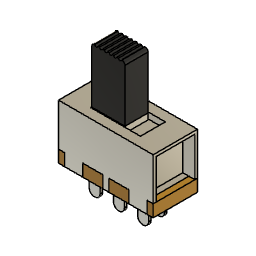
Slide_Switch_SS22F25-G7_ (Autodesk Fusion 360 design; units mm, degrees)
Autodesk Fusion 360 part; units mm, degrees
sketch "Sketch1" plane through (0, 0, 0) normal (0, 1, 0) x (1, 0, 0)
  line L0 (0, 0) -> (15.6, 0)
  line L1 (15.6, 0) -> (15.6, -2)
  line L2 (0, -2) -> (0, 0)
  line L3 (15.6, -2) -> (15.6, -9)
  line L4 (15.6, -9) -> (0, -9)
  line L5 (0, -9) -> (0, -2)
  line L6 (0, -2) -> (1, -2)
  line L7 (1, -2) -> (1, 0)
  line L8 (1, 0) -> (0, 0)
  line L9 (0, 0) -> (0, -2)
  line L10 (15.6, -2) -> (14.6, -2)
  line L11 (14.6, -2) -> (14.6, 0)
  line L12 (14.6, 0) -> (15.6, 0)
  line L13 (15.6, 0) -> (15.6, -2)
  line L14 (11.6, -2) -> (11.6, 0)
  line L15 (11.6, 0) -> (14.6, 0)
  line L16 (14.6, 0) -> (14.6, -2)
  line L17 (4, -2) -> (4, 0)
  line L18 (4, 0) -> (1, 0)
  line L19 (1, 0) -> (1, -2)
  line L20 (7.8, -14) -> (7.8, 4) construction
  line L21 (1, -2) -> (0, -2)
  line L22 (0, -2) -> (1, -2)
  line L23 (15.6, -2) -> (14.6, -2)
  line L24 (14.6, -2) -> (15.6, -2)
  line L25 (8.3, -2) -> (8.3, 0)
  line L26 (8.3, 0) -> (7.3, 0)
  line L27 (7.3, 0) -> (7.3, -2)
  line L28 (4, -2) -> (7.3, -2)
  line L29 (8.3, -2) -> (11.6, -2)
  line L30 (11.6, -2) -> (8.3, -2)
  line L31 (7.3, -2) -> (4, -2)
  dimension "d2" = 2
  dimension "d3" = 15.6
  dimension "d4" = 7
  dimension "d5" = 1
  dimension "d6" = 1
  dimension "d7" = 2
  dimension "d8" = 3
  dimension "d9" = 2
  dimension "d10" = 3
  dimension "d11" = 2
  dimension "d12" = 7.8
  dimension "d13" = 1
  dimension "d14" = 2
  constraint horizontal L0
  constraint vertical L1
  constraint horizontal L23
  constraint vertical L2
  constraint coincident L0.start L2.end
  constraint horizontal L22
  constraint vertical L3
  constraint horizontal L4
  constraint vertical L5
  constraint horizontal L6
  constraint vertical L7
  constraint horizontal L8
  constraint vertical L9
  constraint coincident L0 L7.end
  constraint horizontal L10
  constraint vertical L11
  constraint horizontal L12
  constraint vertical L13
  constraint vertical L14
  constraint horizontal L15
  constraint vertical L16
  constraint vertical L17
  constraint horizontal L18
  constraint vertical L19
  constraint vertical L20
  constraint collinear L21 L23
  constraint collinear L22 L28
  constraint collinear L23 L30
  constraint collinear L24 L28
  constraint vertical L25
  constraint horizontal L26
  constraint vertical L27
  constraint coincident L27.end L30
  constraint collinear L28 L29
  constraint collinear L30 L31
  measures "d2" distance of L0.start L2.start
  measures "d3" distance of L2.start L1.end
  measures "d4" distance of L2.start L4.end
  measures "d5" distance of L2.start L6.end
  measures "d6" distance of L1.end L10.end
  measures "d7" distance of L1.end L0.end
  measures "d8" distance of L10.end L14.start
  measures "d9" distance of L10.end L11.end
  measures "d10" distance of L6.end L17.start
  measures "d11" distance of L6.end L7.end
  measures "d12" distance of L5 L20
  measures "d13" distance of L27.end L25.start
  measures "d14" distance of L27.end L26.end
extrude "Extrude1" add sketch "Sketch1" along normal blind 7.3 contours L0 L3 L4 L5 L6 L7 L10 L11 L14 L15 L16 L17 L18 L19 L21 L22 L23 L24 L25 L26 L27 L28 L29 L30 L31 makes body 1
extrude "Extrude2" add sketch "Sketch1" along normal blind 7.3 separate body contours L0 L2 L6 L7 L8 L9 L19 L21 L22 | L0 L17 L27 L28 L31 | L0 L14 L25 L29 L30 | L0 L1 L10 L11 L12 L13 L16 L23 L24 makes body 2 at (5.1, 2.4333, 0) makes body 3 at (9.4, 2.4333, 0) makes body 4 at (1, 2.4333, 1.3333) makes body 5 at (14.6, 2.4333, 1.3333)
sketch "Sketch2" plane through (0, 0, 9) normal (0, 0, 1) x (-1, 0, 0)
  line L0 (0, 0) -> (-15.6, 0)
  line L1 (-15.6, 0) -> (-15.6, -7.3)
  line L2 (-15.6, -7.3) -> (0, -7.3)
  line L3 (0, -7.3) -> (0, 0)
  line L4 (0, 0) -> (-15.6, -7.3) construction
  line L5 (-15.6, 0) -> (0, -7.3) construction
  line L6 (-11.9, -1.6) -> (-3.7, -1.6)
  line L7 (-3.7, -1.6) -> (-3.7, -5.7)
  line L8 (-3.7, -5.7) -> (-11.9, -5.7)
  line L9 (-11.9, -5.7) -> (-11.9, -1.6)
  line L10 (-11.9, -1.6) -> (-3.7, -5.7) construction
  line L11 (-3.7, -1.6) -> (-11.9, -5.7) construction
  line L12 (-3.7, -5.55) -> (-9.2, -5.55)
  line L13 (-9.2, -5.55) -> (-9.2, -1.75)
  line L14 (-9.2, -1.75) -> (-3.7, -1.75)
  line L15 (-3.7, -1.75) -> (-3.7, -5.55)
  line L16 (1.4148, -3.65) -> (-17, -3.65) construction
  line L17 (1.4148, -1.75) -> (-17, -1.75) construction
  line L18 (-3.7, -1.75) -> (-3.77, -1.75) construction
  point P0 (-7.8, -3.65)
  dimension "d19" = 8.2
  dimension "d20" = 4.1
  dimension "d21" = 5.5
  dimension "d22" = 3.8
  dimension "d23" = 1.9
  constraint coincident L0.start L3.end
  constraint coincident L1.end L2.start
  constraint coincident L0.end L1.start
  constraint coincident L2.end L3.start
  constraint horizontal L6
  constraint perpendicular L6 L7
  constraint parallel L6 L8
  constraint parallel L7 L9
  constraint coincident L10 P0
  constraint coincident L11 P0
  constraint midpoint L5 P0
  constraint horizontal L12
  constraint vertical L13
  constraint horizontal L14
  constraint vertical L15
  constraint perpendicular L1 L16
  constraint coincident L17 L14.end
  constraint coincident L7 L14.end
  constraint coincident L17 L18.end
  measures "d19" distance of L7.end L8.end
  measures "d20" distance of L6.end L7.end
  measures "d21" distance of L12.start L12.end
  measures "d22" distance of L12.start L14.end
extrude "Extrude3" add sketch "Sketch2" along normal blind 9.2 separate body contours L7 L12 L13 L14 L15 makes body 6
extrude "Extrude4" cut sketch "Sketch2" against normal blind 1 contours L6 L7 L8 L9 L12 L13 L14 bodies 1
fillet "Fillet1" radius 0.5 2 edges at (9.2, 3.65, 18.2) (3.7, 3.65, 18.2) on bodies 6
sketch "Sketch3" plane through (0, 1.75, 0) normal (0, -1, 0) x (1, 0, 0)
  arc A0 (4.2, 18.2) -> (3.7, 17.7) centre (4.2, 17.7) ccw
  line L0 (3.7, 17.7) -> (3.7, 9)
  line L1 (3.7, 9) -> (9.2, 9)
  line L2 (9.2, 9) -> (9.2, 17.7)
  arc A1 (9.2, 17.7) -> (8.7, 18.2) centre (8.7, 17.7) ccw
  line L3 (8.7, 18.2) -> (4.2, 18.2)
  circle A2 centre (4.5, 18.2) radius 0.25
  circle A3 centre (5.28, 18.2) radius 0.25
  circle A4 centre (6.06, 18.2) radius 0.25
  circle A5 centre (6.84, 18.2) radius 0.25
  circle A6 centre (7.62, 18.2) radius 0.25
  circle A7 centre (8.4, 18.2) radius 0.25
  dimension "d30" = 0.5
  dimension "d43" = 3.9
  dimension "d44" = 0
  constraint coincident L3 A2.centre
  measures "d30" diameter of A2
extrude "Extrude6" cut sketch "Sketch3" against normal blind 5 contours L3 A2 | L3 A3 | L3 A4 | L3 A7 | L3 A5 | L3 A6 picked at (4.5053, 18.1045) picked at (5.2853, 18.1045) picked at (6.0653, 18.1045) picked at (8.4053, 18.1045) picked at (6.8453, 18.1045) picked at (7.6253, 18.1045) bodies 6
sketch "Sketch4" plane through (15.6, 0, 0) normal (1, 0, 0) x (0, 1, 0)
  line L0 (0, 9) -> (0, 2)
  line L1 (0, 2) -> (7.3, 2)
  line L2 (7.3, 2) -> (7.3, 9)
  line L3 (7.3, 9) -> (0, 9)
  line L4 (0.5, 8.5) -> (6.8816, 8.5)
  line L5 (6.8816, 8.5) -> (6.8816, 2)
  line L6 (6.8816, 2) -> (0.5, 2)
  line L7 (0.5, 2) -> (0.5, 8.5)
  dimension "d47" = 6.5
  constraint horizontal L4
  constraint vertical L5
  constraint horizontal L6
  constraint vertical L7
  measures "d47" distance of L4.start L6.end
extrude "Extrude7" cut sketch "Sketch4" against normal blind 2 contours L1 L4 L5 L6 L7 bodies 1
sketch "Sketch5" plane through (0, 0, 0) normal (-1, 0, 0) x (0, -1, 0)
  line L0 (0, 2) -> (0, 9)
  line L1 (0, 9) -> (-7.3, 9)
  line L2 (-7.3, 9) -> (-7.3, 2)
  line L3 (-7.3, 2) -> (0, 2)
  line L4 (-0.5, 8.5) -> (-6.8462, 8.5)
  line L5 (-6.8462, 8.5) -> (-6.8462, 2)
  line L6 (-6.8462, 2) -> (-0.5, 2)
  line L7 (-0.5, 2) -> (-0.5, 8.5)
  dimension "d50" = 6.5
  constraint horizontal L4
  constraint vertical L5
  constraint horizontal L6
  constraint vertical L7
  measures "d50" distance of L4.start L6.end
extrude "Extrude8" cut sketch "Sketch5" against normal blind 2 contours L3 L4 L5 L6 L7 bodies 1
sketch "Sketch6" plane through (0, 0, 0) normal (0, 0, -1) x (1, 0, 0)
  line L0 (7.3, 0) -> (4, 0)
  line L1 (4, 0) -> (4, -7.3)
  line L2 (4, -7.3) -> (7.3, -7.3)
  line L3 (7.3, -7.3) -> (7.3, 0)
  line L4 (11.8, -2.35) -> (3.8, -2.35) construction
  line L5 (3.8, -2.35) -> (3.8, -4.95) construction
  line L6 (3.8, -4.95) -> (11.8, -4.95) construction
  line L7 (11.8, -4.95) -> (11.8, -2.35) construction
  line L8 (11.8, -2.35) -> (3.8, -4.95) construction
  line L9 (3.8, -2.35) -> (11.8, -4.95) construction
  line L10 (7.8, 2) -> (7.8, -8.6458) construction
  line L11 (4.7, -2.15) -> (2.9, -2.15)
  line L12 (2.9, -2.15) -> (2.9, -2.55)
  line L13 (2.9, -2.55) -> (4.7, -2.55)
  line L14 (4.7, -2.55) -> (4.7, -2.15)
  line L15 (4.7, -2.15) -> (2.9, -2.55) construction
  line L16 (2.9, -2.15) -> (4.7, -2.55) construction
  line L17 (4.7, -5.15) -> (2.9, -5.15)
  line L18 (2.9, -5.15) -> (2.9, -4.75)
  line L19 (2.9, -4.75) -> (4.7, -4.75)
  line L20 (4.7, -4.75) -> (4.7, -5.15)
  line L21 (4.7, -5.15) -> (2.9, -4.75) construction
  line L22 (2.9, -5.15) -> (4.7, -4.75) construction
  line L23 (8.7, -2.55) -> (6.9, -2.55)
  line L24 (6.9, -2.55) -> (6.9, -2.15)
  line L25 (6.9, -2.15) -> (8.7, -2.15)
  line L26 (8.7, -2.15) -> (8.7, -2.55)
  line L27 (8.7, -2.55) -> (6.9, -2.15) construction
  line L28 (6.9, -2.55) -> (8.7, -2.15) construction
  line L29 (8.7, -5.15) -> (6.9, -5.15)
  line L30 (6.9, -5.15) -> (6.9, -4.75)
  line L31 (6.9, -4.75) -> (8.7, -4.75)
  line L32 (8.7, -4.75) -> (8.7, -5.15)
  line L33 (8.7, -5.15) -> (6.9, -4.75) construction
  line L34 (6.9, -5.15) -> (8.7, -4.75) construction
  line L35 (12.7, -2.55) -> (10.9, -2.55)
  line L36 (10.9, -2.55) -> (10.9, -2.15)
  line L37 (10.9, -2.15) -> (12.7, -2.15)
  line L38 (12.7, -2.15) -> (12.7, -2.55)
  line L39 (12.7, -2.55) -> (10.9, -2.15) construction
  line L40 (10.9, -2.55) -> (12.7, -2.15) construction
  line L41 (12.7, -5.15) -> (10.9, -5.15)
  line L42 (10.9, -5.15) -> (10.9, -4.75)
  line L43 (10.9, -4.75) -> (12.7, -4.75)
  line L44 (12.7, -4.75) -> (12.7, -5.15)
  line L45 (12.7, -5.15) -> (10.9, -4.75) construction
  line L46 (10.9, -5.15) -> (12.7, -4.75) construction
  point P0 (7.8, -3.65)
  point P1 (3.8, -2.35)
  point P2 (3.8, -4.95)
  point P3 (7.8, -2.35)
  point P4 (7.8, -4.95)
  point P5 (11.8, -2.35)
  point P6 (11.8, -4.95)
  dimension "d53" = 8
  dimension "d54" = 2.6
  dimension "d55" = 1.8
  dimension "d56" = 0.4
  dimension "d57" = 1.8
  dimension "d58" = 0.4
  dimension "d59" = 1.8
  dimension "d60" = 0.4
  dimension "d61" = 1.8
  dimension "d62" = 0.4
  dimension "d63" = 1.8
  dimension "d64" = 0.4
  dimension "d65" = 1.8
  dimension "d66" = 0.4
  constraint horizontal L4
  constraint perpendicular L4 L5
  constraint parallel L4 L6
  constraint parallel L5 L7
  constraint coincident L8 P0
  constraint coincident L9 P0
  constraint parallel L3 L10
  constraint horizontal L11
  constraint perpendicular L11 L12
  constraint parallel L11 L13
  constraint parallel L12 L14
  constraint coincident L15 P1
  constraint coincident L16 P1
  constraint coincident P1 L4.end
  constraint horizontal L17
  constraint perpendicular L17 L18
  constraint parallel L17 L19
  constraint parallel L18 L20
  constraint coincident L21 P2
  constraint coincident L22 P2
  constraint coincident P2 L5.end
  constraint horizontal L23
  constraint perpendicular L23 L24
  constraint parallel L23 L25
  constraint parallel L24 L26
  constraint coincident L27 P3
  constraint coincident L28 P3
  constraint midpoint L4 P3
  constraint horizontal L29
  constraint perpendicular L29 L30
  constraint parallel L29 L31
  constraint parallel L30 L32
  constraint coincident L33 P4
  constraint coincident L34 P4
  constraint midpoint L6 P4
  constraint horizontal L35
  constraint perpendicular L35 L36
  constraint parallel L35 L37
  constraint parallel L36 L38
  constraint coincident L39 P5
  constraint coincident L40 P5
  constraint coincident L4.start L7.end
  constraint horizontal L41
  constraint perpendicular L41 L42
  constraint parallel L41 L43
  constraint parallel L42 L44
  constraint coincident L45 P6
  constraint coincident L46 P6
  constraint coincident P6 L6.end
  measures "d53" distance of P2 P6
  measures "d54" distance of P1 P2
  measures "d55" distance of L12.end L13.end
  measures "d56" distance of L11.end L12.end
  measures "d57" distance of L18.end L19.end
  measures "d58" distance of L17.end L18.end
  measures "d59" distance of L24.end L25.end
  measures "d60" distance of L23.end L24.end
  measures "d61" distance of L30.end L31.end
  measures "d62" distance of L29.end L30.end
  measures "d63" distance of L36.end L37.end
  measures "d64" distance of L35.end L36.end
  measures "d65" distance of L42.end L43.end
  measures "d66" distance of L41.end L42.end
extrude "Extrude9" add sketch "Sketch6" along normal blind 4 separate body contours L3 L23 L25 L26 | L3 L23 L24 L25 | L1 L11 L13 L14 | L1 L11 L12 L13 | L3 L29 L31 L32 | L3 L29 L30 L31 | L1 L17 L19 L20 | L1 L17 L18 L19 | L35 L36 L37 L38 | L41 L42 L43 L44 makes body 7 at (7.5, 4.75, -1.3333) makes body 8 at (4.1, 2.15, -1.3333) makes body 9 at (12.1, 2.55, -1.3333) makes body 10 at (7.5, 2.15, -1.3333) makes body 11 at (3.5, 4.75, -1.3333) makes body 12 at (12.1, 5.15, -1.3333)
fillet "Fillet2" radius 0.9 12 edges at (6.9, 4.95, -4) (8.7, 4.95, -4) (2.9, 2.35, -4) (4.7, 2.35, -4) (10.9, 2.35, -4) (12.7, 2.35, -4) (6.9, 2.35, -4) (8.7, 2.35, -4) (2.9, 4.95, -4) (4.7, 4.95, -4) (10.9, 4.95, -4) (12.7, 4.95, -4) on bodies 7 8 9 10 11 12
